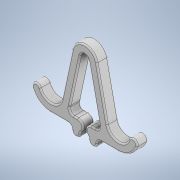
# Autodesk Inventor part: DoubleBedDowelHook
Saved by Autodesk Inventor 2020 (Build 240168000, 168)
## iProperties
Created: 2019-12-18
Part Number: DoubleBedDowelHook
Material: Generic
Document SubType Name: Modeling
Designer: Connor
Density: 1 g/cm^3
Appearance: Default
Author: Connor
Autodesk Inventor part; units mm, degrees
ref_plane "YZ Plane" through (0, 0, 0) normal (1, 0, 0) x (0, 1, 0)
ref_plane "XZ Plane" through (0, 0, 0) normal (0, 1, 0) x (-1, 0, 0)
ref_plane "XY Plane" through (0, 0, 0) normal (0, 0, 1) x (1, 0, 0)
sketch "Sketch2" plane through (0, 0, 0) normal (0, 0, 1) x (1, 0, 0)
  circle A0 centre (0, 0) radius 4.7625
  circle A1 centre (0, -76.2) radius 4.7625
  circle A2 centre (0, 0) radius 14.2875 construction
  circle A3 centre (0, -76.2) radius 14.2875 construction
  circle A4 centre (38.1, -49.2125) radius 12.7 construction
  circle A5 centre (9.525, 0) radius 4.7625 construction
  line L0 (-38.1, -61.9125) -> (0, -61.9125) construction
  circle A6 centre (-38.1, -49.2125) radius 12.7 construction
  line L1 (0, -61.9125) -> (38.1, -61.9125) construction
  arc A7 (13.9727, 2.9825) -> (-13.9727, 2.9825) centre (0, 0) ccw
  line L2 (-25.6798, -51.8636) -> (-13.9727, 2.9825)
  line L3 (13.9727, 2.9825) -> (25.6798, -51.8636)
  circle A8 centre (-54.5094, -55.185) radius 4.7625
  circle A9 centre (54.5094, -55.185) radius 4.7625
  arc A10 (-50.0341, -53.5562) -> (-25.6798, -51.8636) centre (-38.1, -49.2125) ccw
  line L4 (-38.1, -49.2125) -> (-25.4, -49.2125) construction
  line L5 (-38.1, -49.2125) -> (-50.0341, -53.5562) construction
  arc A11 (25.6798, -51.8636) -> (50.0341, -53.5562) centre (38.1, -49.2125) ccw
  line L6 (38.1, -49.2125) -> (50.0341, -53.5562) construction
  line L7 (38.1, -49.2125) -> (25.4, -49.2125) construction
  arc A12 (-58.9847, -56.8139) -> (-16.3646, -53.852) centre (-38.1, -49.2125) ccw
  line L8 (-16.3646, -53.852) -> (-4.6576, 0.9942)
  line L9 (16.3646, -53.852) -> (4.6576, 0.9942)
  circle A13 centre (9.525, -76.2) radius 4.7625
  circle A14 centre (-9.525, -76.2) radius 4.7625
  line L10 (-38.1, -71.4375) -> (-9.525, -71.4375)
  arc A15 (16.3646, -53.852) -> (58.9847, -56.8139) centre (38.1, -49.2125) ccw
  line L11 (9.525, -71.4375) -> (38.1, -71.4375)
  arc A16 (-14.2875, -76.2) -> (-19.05, -71.4375) centre (-19.05, -76.2) ccw
  arc A17 (19.05, -71.4375) -> (14.2875, -76.2) centre (19.05, -76.2) ccw
  line L12 (-19.861, -61.9125) -> (19.861, -61.9125)
  arc A18 (-16.858, -55.7493) -> (-12.3062, -61.9125) centre (-12.3062, -57.15) ccw
  arc A19 (12.3062, -61.9125) -> (16.858, -55.7493) centre (12.3062, -57.15) ccw
  point P0 (-4.7625, -76.2)
  point P1 (4.7625, -76.2)
  point P2 (14.2875, -76.2)
  dimension "d18" = 9.525
  dimension "d19" = 76.2
  dimension "d20" = 76.2
  dimension "d21" = 25.4
  dimension "d23" = 160
  dimension "d24" = 160
  constraints: 43 point on circle, 27 tangent, 26 end point, 18 centre point, 11 equal radius, 8 coincident, 8 point on line, 6 horizontal, 3 horizontal alignment, 1 collinear, 1 concentric, 1 vertical alignment, 12 other
  measures "d18" diameter of A0
  measures "d19" distance of A1.centre point (0, 0)
  measures "d20" distance of A4.centre A6.centre
  measures "d21" diameter of A4
  measures "d23" angle of L5 L4
  measures "d24" angle of L7 L6
extrude "Extrusion2" add sketch "Sketch2" along normal blind 12.7 contours A0 L8 A12 A8 A10 L2 A7 L3 A11 A9 A15 L9 | A15 L12 A19 | A18 L12 A12 | A15 L11 A13 A1 A14 L10 A12 L12 | A9 | A17 A13 L11 | A8 | L10 A14 A16 | A13 | A14
sketch "Sketch4" plane through (0, 0, 12.7) normal (0, 0, 1) x (1, 0, 0)
  arc A0 (-14.2875, -76.2) -> (-4.7625, -76.2) centre (-9.525, -76.2) ccw projected
  arc A1 (4.7625, -76.2) -> (14.2875, -76.2) centre (9.525, -76.2) ccw projected
  arc A2 (58.9847, -56.8139) -> (50.0341, -53.5562) centre (54.5094, -55.185) ccw projected
  arc A3 (25.6798, -51.8636) -> (50.0341, -53.5562) centre (38.1, -49.2125) ccw projected
  line L0 (25.6798, -51.8636) -> (13.9727, 2.9825) projected
  arc A4 (13.9727, 2.9825) -> (-13.9727, 2.9825) centre (0, 0) ccw projected
  line L1 (-13.9727, 2.9825) -> (-25.6798, -51.8636) projected
  arc A5 (-50.0341, -53.5562) -> (-25.6798, -51.8636) centre (-38.1, -49.2125) ccw projected
  arc A6 (-50.0341, -53.5562) -> (-58.9847, -56.8139) centre (-54.5094, -55.185) ccw projected
  arc A7 (-58.9847, -56.8139) -> (-38.1, -71.4375) centre (-38.1, -49.2125) ccw projected
  line L2 (-16.3646, -53.852) -> (-4.6576, 0.9942) projected
  arc A8 (4.6576, 0.9942) -> (-4.6576, 0.9942) centre (0, 0) ccw projected
  line L3 (4.6576, 0.9942) -> (16.3646, -53.852) projected
  circle A9 centre (7.7771, -68.2625) radius 6.35
  circle A10 centre (-7.7771, -68.2625) radius 6.35
  arc A11 (16.3646, -53.852) -> (16.858, -55.7493) centre (38.1, -49.2125) ccw projected
  arc A12 (19.05, -71.4375) -> (14.2875, -76.2) centre (19.05, -76.2) ccw projected
  line L4 (19.05, -71.4375) -> (38.1, -71.4375) projected
  arc A13 (38.1, -71.4375) -> (58.9847, -56.8139) centre (38.1, -49.2125) ccw projected
  line L5 (-38.1, -71.4375) -> (-19.05, -71.4375) projected
  arc A14 (-14.2875, -76.2) -> (-19.05, -71.4375) centre (-19.05, -76.2) ccw projected
  arc A15 (4.7625, -76.2) -> (-4.7625, -76.2) centre (0, -76.2) ccw projected
  arc A16 (-16.858, -55.7493) -> (-16.3646, -53.852) centre (-38.1, -49.2125) ccw projected
  arc A17 (12.3062, -61.9125) -> (16.858, -55.7493) centre (12.3062, -57.15) ccw projected
  line L6 (12.3062, -61.9125) -> (-12.3062, -61.9125) projected
  arc A18 (-16.858, -55.7493) -> (-12.3062, -61.9125) centre (-12.3062, -57.15) ccw projected
  arc A19 (4.7625, -76.2) -> (-4.7625, -76.2) centre (0, -76.2) ccw projected
  point P0 (7.7771, -61.9125)
  point P1 (-7.7771, -61.9125)
  point P2 (-3.3331, -72.7982)
  point P3 (3.3331, -72.7982)
  dimension "d32" = 12.7
  constraints: 4 tangent, 2 centre point, 1 equal radius
  measures "d32" diameter of A10
extrude "Extrusion3" cut sketch "Sketch4" against normal through all contours A10 L6 A9 A15
fillet "Fillet2" radius 1.5875 56 edges at (-37.2195, -61.8819, 12.7) (-56.1383, -50.7097, 12.7) (-50.8477, -67.4182, 12.7) (-28.575, -71.4375, 12.7) (-15.6824, -72.8324, 12.7) (-9.525, -80.9625, 12.7) (-4.3906, -74.355, 12.7) (-1.8982, -65.8624, 12.7) (-10.0417, -61.9125, 12.7) (-16.1371, -59.9793, 12.7) (-16.5904, -54.8061, 12.7) (-10.5111, -26.4289, 12.7) (0, 4.7625, 12.7) (10.5111, -26.4289, 12.7) (16.5904, -54.8061, 12.7) (16.1371, -59.9793, 12.7) (10.0417, -61.9125, 12.7) (1.8982, -65.8624, 12.7) (4.3906, -74.355, 12.7) (9.525, -80.9625, 12.7) (15.6824, -72.8324, 12.7) (28.575, -71.4375, 12.7) (50.8477, -67.4182, 12.7) (56.1383, -50.7097, 12.7) (37.2195, -61.8819, 12.7) (19.8263, -24.4406, 12.7) (0, 14.2875, 12.7) (-19.8263, -24.4406, 12.7) (-37.2195, -61.8819, 0) (-56.1383, -50.7097, 0) (-50.8477, -67.4182, 0) (-28.575, -71.4375, 0) (-15.6824, -72.8324, 0) (-9.525, -80.9625, 0) (-4.3906, -74.355, 0) (-1.8982, -65.8624, 0) (-10.0417, -61.9125, 0) (-16.1371, -59.9793, 0) (-16.5904, -54.8061, 0) (-10.5111, -26.4289, 0) (0, 4.7625, 0) (10.5111, -26.4289, 0) (16.5904, -54.8061, 0) (16.1371, -59.9793, 0) (10.0417, -61.9125, 0) (1.8982, -65.8624, 0) (4.3906, -74.355, 0) (9.525, -80.9625, 0) (15.6824, -72.8324, 0) (28.575, -71.4375, 0) (50.8477, -67.4182, 0) (56.1383, -50.7097, 0) (37.2195, -61.8819, 0) (19.8263, -24.4406, 0) (0, 14.2875, 0) (-19.8263, -24.4406, 0)
body "Solid2"
